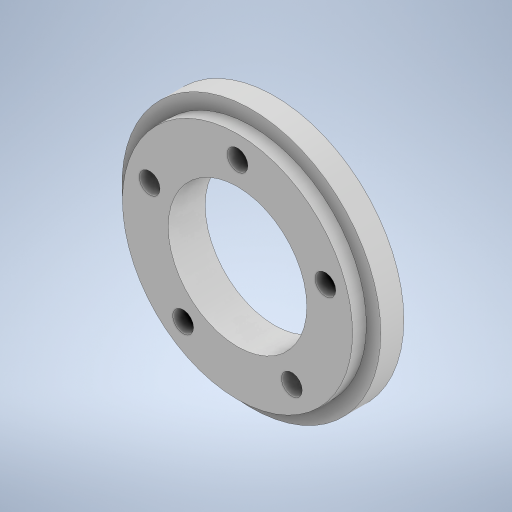
# Autodesk Inventor part: 사이클로이드 기어 축 연결 하우징
Saved by Autodesk Inventor 2023 (Build 270158000, 158)
## iProperties
Created: 2022-06-20
Part Number: 사이클로이드 기어 축 연결 하우징
Material: 일반
Document SubType Name: Modeling
Designer: fly01
Density: 1 g/cm^3
Appearance: 기본값
Author: fly01
Autodesk Inventor part; units mm, degrees
ref_plane "YZ Plane" through (0, 0, 0) normal (1, 0, 0) x (0, 1, 0)
ref_plane "XZ Plane" through (0, 0, 0) normal (0, 1, 0) x (-1, 0, 0)
ref_plane "XY Plane" through (0, 0, 0) normal (0, 0, 1) x (1, 0, 0)
sketch "스케치1" plane through (0, 0, 0) normal (0, 0, 1) x (1, 0, 0)
  circle A0 centre (0, 0) radius 24.9
  circle A1 centre (0, 0) radius 28
  circle A2 centre (0, 0) radius 15
  dimension "d0" = 49.8
  dimension "d1" = 56
  dimension "d2" = 30
  constraints: 3 centre point, 3 coincident
  measures "d0" diameter of A0
  measures "d1" diameter of A1
  measures "d2" diameter of A2
extrude "돌출1" add sketch "스케치1" along normal blind 3 contours A0
extrude "돌출2" add sketch "스케치1" against normal blind 5 contours A0 | A1
sketch "스케치3" plane through (0, 0, 3) normal (0, 0, 1) x (1, 0, 0)
  circle A0 centre (0, 0) radius 20 construction
  circle A1 centre (0, 20) radius 2.25
  circle A2 centre (-19.0211, 6.1803) radius 2.25
  circle A3 centre (-11.7557, -16.1803) radius 2.25
  circle A4 centre (11.7557, -16.1803) radius 2.25
  circle A5 centre (19.0211, 6.1803) radius 2.25
  dimension "d9" = 40
  dimension "d10" = 4.5
  dimension "d13" = 360
  constraints: 5 centre point, 1 coincident, 1 vertical alignment, 13 other
  measures "d10" diameter of A1
extrude "돌출3" cut sketch "스케치3" against normal blind 44.5
